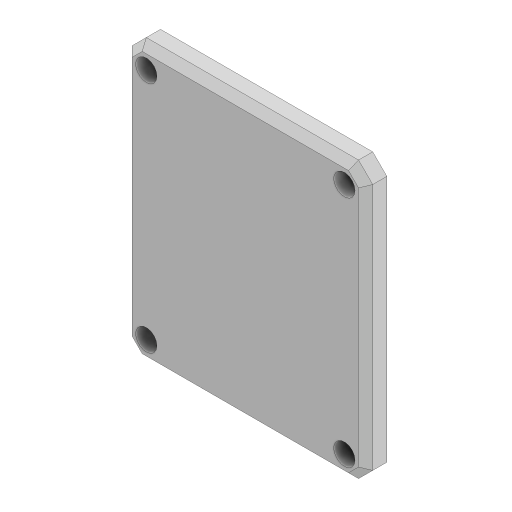
# Autodesk Inventor part: manta ray handle cap
Saved by Autodesk Inventor 2024 (Build 280153000, 153)
## iProperties
Created: 2024-01-12
Part Number: manta ray handle cap
Material: Generic
Document SubType Name: Modeling
Designer: chris
Density: 1 g/cm^3
Appearance: Default
Author: chris
Autodesk Inventor part; units mm, degrees
ref_plane "YZ Plane" through (0, 0, 0) normal (1, 0, 0) x (0, 1, 0)
ref_plane "XZ Plane" through (0, 0, 0) normal (0, 1, 0) x (-1, 0, 0)
ref_plane "XY Plane" through (0, 0, 0) normal (0, 0, 1) x (1, 0, 0)
sketch "Sketch1" plane through (0, 0, 0) normal (0, 0, 1) x (1, 0, 0)
  circle A0 centre (-14, 16.5) radius 1.5
  circle A1 centre (14, 16.5) radius 1.5
  line L0 (-12, 0) -> (-12, 14.5)
  line L1 (-12, 14.5) -> (12, 14.5)
  line L2 (12, 14.5) -> (12, 0)
  line L3 (12, 0) -> (17, 0)
  line L4 (17, 0) -> (17, 17.5)
  line L5 (15, 19.5) -> (17, 17.5)
  line L6 (-15, 19.5) -> (15, 19.5)
  line L7 (-17, 17.5) -> (-15, 19.5)
  line L8 (-17, 0) -> (-17, 17.5)
  line L9 (-17, 0) -> (-12, 0)
  line L10 (0, 14.5) -> (0, 0)
  circle A2 centre (-14, -16.5) radius 1.5
  circle A3 centre (14, -16.5) radius 1.5
  line L11 (-12, 0) -> (-12, -14.5)
  line L12 (-12, -14.5) -> (12, -14.5)
  line L13 (12, -14.5) -> (12, 0)
  line L14 (17, 0) -> (17, -17.5)
  line L15 (15, -19.5) -> (17, -17.5)
  line L16 (-15, -19.5) -> (15, -19.5)
  line L17 (-17, -17.5) -> (-15, -19.5)
  line L18 (-17, 0) -> (-17, -17.5)
  line L19 (0, -14.5) -> (0, 0)
  point P0 (0, 0)
  point P1 (0, 12)
  point P2 (0, -12)
  constraints: 40 end point, 10 symmetric about line, 4 centre point, 1 midpoint, 1 vertical, 2 other
extrude "Extrusion1" add sketch "Sketch1" along normal blind 3
chamfer "Chamfer1" distance 1 angle 45 8 edges at (-16, -18.5, 3) (-16, 18.5, 3) (16, 18.5, 3) (16, -18.5, 3) (0, -19.5, 3) (0, 19.5, 3) (-17, 8.75, 3) (17, 8.75, 3)
body "Solid1"
